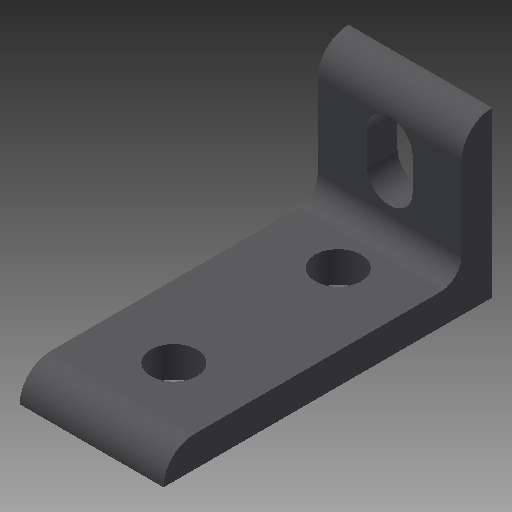
# Autodesk Inventor part: 4250
Saved by Autodesk Inventor 2017 (Build 210142000, 142)
## iProperties
Category: PARTsolutions
Company: 8020
Created: 2017-04-25
Part Number: 4250
Catalog Web Link: www.cadenas.de
Description: 4250, 4280-Joining Plates - 3 Hole Slotted Inside Corner Bracket
Vendor: 8020
Document SubType Name: Modeling
Designer: psAdmin
Manufacturer: 8020
Mass: 6.64346 g
Surface Area: 39.8651 cm^2
Volume: 6.64346 cm^3
Density: 1 g/cm^3
Material: Generic
Appearance: PSOLRGB-175-175-175
PSOL_IDENT_0: {$CADENAS_DATA\23d-libs\8020\inch\joining_plates\4250.prj},145 {VTYP=3D},{NB=4250},{LINA=4250},{NN=4
PSOL_IDENT_1: 250, 4280},{DATE=22.08.2012},{GEOMDATE=07.12.2011 07:37:00},{VERSION=},{LINEID=10},{LINESUBID=-1},{W
PSOL_IDENT_2: BVAR=}  {NB=4250},{LINA=4250},{KT=DUMMY},{PN=4250},{A=0.875},{B=2.000},{C=1.000},{D=0.312},{E=0.188}
PSOL_IDENT_3: ,{F=0.281},{W=.040},{A1=0.500},{A2=1.500},{D1=0.187},{R=0.125}
NN: 4250, 4280
NT: Joining Plates - 3 Hole Slotted Inside Corner Bracket
NB: 4250
NBSYN: $PN.
LINA: 4250
PN: 4250
A: 0.875
B: 2.000
C: 1.000
D: 0.312
E: 0.188
F: 0.281
W: .040
SUPPLIER: 8020
ARTICLENO: 4250
BOMINFO: 4250
CREATOR: CADENAS GmbH
Title: 4250
Author: Cadenas PARTsolutions
Comments: Joining Plates - 3 Hole Slotted Inside Corner Bracket
Autodesk Inventor part; units mm, degrees
ref_plane "YZ Plane" through (0, 0, 0) normal (1, 0, 0) x (0, 1, 0)
ref_plane "XZ Plane" through (0, 0, 0) normal (0, 1, 0) x (-1, 0, 0)
ref_plane "XY Plane" through (0, 0, 0) normal (0, 0, 1) x (1, 0, 0)
sketch "Sketch_1" plane through (0, 0, 0) normal (1, 0, 0) x (0, 1, 0)
  line L0 (0, 50.8) -> (0, 0)
  line L1 (0, 0) -> (25.4, 0)
  arc A0 (25.4, 0) -> (20.6502, 4.7498) centre (20.6502, 0) ccw
  line L2 (20.6502, 4.7498) -> (7.9248, 4.7498)
  arc A1 (4.7498, 7.9248) -> (7.9248, 4.7498) centre (7.9248, 7.9248) ccw
  line L3 (4.7498, 7.9248) -> (4.7498, 46.0502)
  arc A2 (4.7498, 46.0502) -> (0, 50.8) centre (0, 46.0502) ccw
  constraints: 8 end point, 6 point on circle, 3 centre point
extrude "Extrusion1" add sketch "Sketch_1" along normal mid plane 22.225
sketch "Sketch_2" plane through (0, 0, 0) normal (0, 0, 1) x (1, 0, 0)
  arc A0 (-3.5687, 12.7) -> (3.5687, 12.7) centre (0, 12.7) ccw
  line L0 (3.5687, 12.7) -> (3.5687, 17.4752)
  arc A1 (3.5687, 17.4752) -> (-3.5687, 17.4752) centre (0, 17.4752) ccw
  line L1 (-3.5687, 17.4752) -> (-3.5687, 12.7)
  constraints: 4 end point, 4 point on circle, 2 centre point
extrude "Extrusion2" cut sketch "Sketch_2" along normal blind 7.9248
sketch "Sketch3" plane through (-11.1125, 0, 50.8) normal (0, -1, 0) x (1, 0, 0)
  point P0 (11.1125, -38.1)
hole "Hole1" at (0, 0, 12.7) direction (0, 1, 0) diameter 7.1374 depth 7.9248
sketch "Sketch4" plane through (-11.1125, 0, 50.8) normal (0, -1, 0) x (1, 0, 0)
  point P0 (11.1125, -12.7)
hole "Hole2" at (0, 0, 38.1) direction (0, 1, 0) diameter 7.1374 depth 7.9248
body "Solid1"
